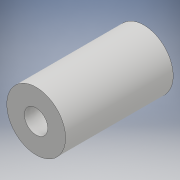
# Autodesk Inventor part: Деталь2
Saved by Autodesk Inventor 2018.1 (Build 221171000, 171)
## iProperties
Created: 2023-04-03
Part Number: Деталь2
Material: Типовые
Document SubType Name: Modeling
Designer: student
Density: 1 g/cm^3
Appearance: По умолчанию
Author: student
Autodesk Inventor part; units mm, degrees
ref_plane "YZ Plane" through (0, 0, 0) normal (1, 0, 0) x (0, 1, 0)
ref_plane "XZ Plane" through (0, 0, 0) normal (0, 1, 0) x (-1, 0, 0)
ref_plane "XY Plane" through (0, 0, 0) normal (0, 0, 1) x (1, 0, 0)
sketch "Эскиз1" plane through (0, 0, 0) normal (0, 1, 0) x (-1, 0, 0)
  circle A0 centre (0, 0) radius 15
  dimension "d0" = 30
  constraints: 1 centre point, 1 coincident
  measures "d0" diameter of A0
extrude "Выдавливание1" add sketch "Эскиз1" along normal blind 55
hole "Отверстие1" at (-0.0551, 55, -0.1504) direction (0, -1, 0) diameter 12 depth 55 tip angle 118
hole "Отверстие2" at (0.0739, 55, -0.1164) direction (0, -1, 0) diameter 20 depth 25 tip angle 118
thread "Резьба1" size "M20x2.5" class "6H" standard "ANSI Metric M Profile" length 20
chamfer "Фаска1" distance 2 angle 45 1 edges at (0.0739, 55, -10.1164)
